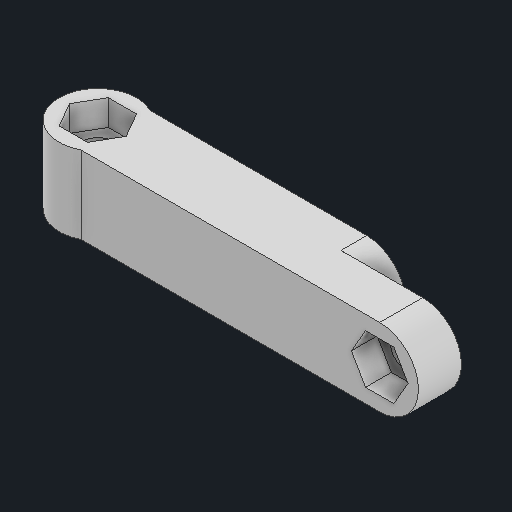
# Autodesk Inventor part: L1
Saved by Autodesk Inventor 2023.4 (Build 274418000, 418)
## iProperties
Created: 2024-10-16
Part Number: L1
Material: Ogólny
Document SubType Name: Modeling
Designer: kamil
Density: 1 g/cm^3
Appearance: Domyślna
Author: kamil
Autodesk Inventor part; units mm, degrees
ref_plane "YZ Plane" through (0, 0, 0) normal (1, 0, 0) x (0, 1, 0)
ref_plane "Płaszczyzna konstrukcyjna2" through (-16.0063, -4.5, 5) normal (0, 0, 1) x (1, 0, 0)
sketch "Szkic1" plane through (0, 0, 0) normal (0, 0, 1) x (1, 0, 0)
  circle A0 centre (-21, 0) radius 1.75 projected
  arc A1 (-11.0125, 4.5) -> (-15.9781, 0.0856) centre (-11.0125, -0.5) ccw projected
  line L0 (-21, 4.5) -> (-11.0125, 4.5) projected
  arc A2 (-21, 4.5) -> (-21, -4.5) centre (-21, 0) ccw projected
  line L1 (-11.0628, -4.5) -> (-21, -4.5) projected
  arc A3 (-15.9446, -0.5811) -> (-11.0628, -4.5) centre (-11.0628, 0.5) ccw projected
  line L2 (-21, 0) -> (-57.75, 0)
  line L3 (-21, 0) -> (-57.75, 0) construction
  line L4 (-21, -4.5) -> (-57.75, -4.5)
  line L5 (-57.75, 4.5) -> (-21, 4.5)
  arc A4 (-21, -4.5) -> (-21, 4.5) centre (-21, 0) ccw
  arc A5 (-57.75, 4.5) -> (-57.75, -4.5) centre (-57.75, 0) ccw
  line L6 (-57.75, 4.5) -> (-57.75, -4.5)
  arc A6 (-15.9781, 0.0856) -> (-15.9446, -0.5811) centre (-13.9919, -0.1486) ccw projected
  point P0 (0, 0)
  point P1 (-39.375, 0)
  dimension "d0" = 36.75
  constraints: 12 end point, 4 point on circle, 4 tangent, 2 centre point, 2 parallel, 1 collinear, 1 midpoint, 1 vertical
  measures "d0" distance of L2.start L2.end
extrude "Wyciągnięcie proste1" add sketch "Szkic1" along normal up to surface (5 mm away) contours A2 A4 | A2 L4 L6 L2 | L2 L6 L5 A2
sketch "Szkic2" plane through (0, 0, 0) normal (0, 0, -1) x (-1, 0, 0)
  line L0 (21, 4.5) -> (57.75, 4.5) projected
  arc A0 (21, 4.5) -> (21, -4.5) centre (21, 0) ccw projected
  line L1 (57.75, -4.5) -> (21, -4.5) projected
  line L2 (57.75, 4.5) -> (57.75, -4.5) projected
  circle A1 centre (21, 0) radius 1.75 projected
  arc A2 (21, -4.5) -> (21, 4.5) centre (21, 0) ccw projected
  circle A3 centre (21, 0) radius 5
  point P0 (0, 0)
  point P1 (23.1794, 4.5)
  point P2 (23.1794, -4.5)
  dimension "d3" = 10
  constraints: 1 centre point, 1 coincident
  measures "d3" diameter of A3
ref_plane "Płaszczyzna konstrukcyjna1" through (-25.5, -4.5, -3) normal (0, 0, -1) x (0, 1, 0)
extrude "Wyciągnięcie proste2" add sketch "Szkic2" along normal up to surface (3 mm away) contours L0 L2 L1 A3
fillet "Zaokrąglenie1" radius 4.5 2 edges at (-23.1794, -4.5, -1.5) (-23.1794, 4.5, -1.5)
sketch "Szkic4" plane through (-57.75, 4.5, 5) normal (0, 1, 0) x (1, 0, 0)
  line L0 (0, 8) -> (0, 0) projected
  circle A0 centre (0, 4) radius 1.75
  circle A1 centre (0, 4) radius 4
  point P0 (57.75, 5)
  point P1 (0, 2.25)
  point P2 (0, 5.75)
  dimension "d15" = 3.5
  constraints: 1 centre point, 1 coincident, 1 midpoint, 3 other
  measures "d15" diameter of A0
extrude "Wyciągnięcie proste6" add sketch "Szkic4" against normal up to surface (9 mm away) contours L0 A0 A1 picked at (-0.4587, 0.8057)
extrude "Wyciągnięcie proste7" cut sketch "Szkic4" against normal through all contours A0 L0 picked at (0.2531, 4.5256)
sketch "Szkic5" plane through (-30.5, 0, -3) normal (0, 0, -1) x (-1, 0, 0)
  arc A0 (0, 4.5) -> (0, -4.5) centre (0, 0) ccw projected
  line L0 (27.25, -4.5) -> (0, -4.5) projected
  line L1 (27.25, 4.5) -> (27.25, -4.5) projected
  line L2 (0, 4.5) -> (27.25, 4.5) projected
  line L3 (29, -4.5) -> (29, 4.5) projected
  line L4 (25.5, -4.5) -> (25.5, 4.5) projected
  line L5 (23.5, -4.5) -> (23.5, 4.5)
  arc A1 (0, 2.5) -> (0, -2.5) centre (0, 0) ccw
  line L6 (0, 2.5) -> (25.25, 2.5)
  line L7 (25.25, 2.5) -> (25.25, -2.5)
  line L8 (25.25, -2.5) -> (0, -2.5)
  point P0 (-30.5, 0)
  point P1 (23.5, -2.5)
  point P2 (23.5, 2.5)
  dimension "d20" = 2
  dimension "d21" = 2
  constraints: 8 end point, 2 point on circle, 1 centre point, 1 parallel, 3 other
  measures "d20" distance between parallel lines of L4 L5
  measures "d21" distance between parallel lines of L0 L8
extrude "Wyciągnięcie proste8" cut sketch "Szkic5" against normal up to surface (3 mm away) contours L5 L8 A1 L6
fillet "Zaokrąglenie2" radius 2 2 edges at (-54, 2.5, -1.5) (-54, -2.5, -1.5)
sketch "Szkic6" plane through (-21, 0, 5) normal (0, 0, 1) x (1, 0, 0)
  circle A0 centre (0, 0) radius 1.75 projected
  circle A1 centre (0, 0) radius 2.85
  line L0 (1.6454, 2.85) -> (3.2909, 0)
  line L1 (3.2909, 0) -> (1.6454, -2.85)
  line L2 (1.6454, -2.85) -> (-1.6454, -2.85)
  line L3 (-1.6454, -2.85) -> (-3.2909, 0)
  line L4 (-3.2909, 0) -> (-1.6454, 2.85)
  line L5 (-1.6454, 2.85) -> (1.6454, 2.85)
  point P0 (21, 0)
  point P1 (0, 2.85)
  dimension "d25" = 5.7
  constraints: 12 end point, 2 coincident, 1 midpoint, 1 vertical alignment, 15 other
extrude "Wyciągnięcie proste9" cut sketch "Szkic6" against normal blind 3 contours A0 | A1 | A1 L0 L1 | A1 L5 L0 | L1 L2 A1 | A1 L4 L5 | L2 L3 A1 | A1 L3 L4
sketch "Szkic7" plane through (-21, 4.5, 5) normal (0, 1, 0) x (1, 0, 0)
  circle A0 centre (-36.75, 4) radius 1.75 projected
  circle A1 centre (-36.75, 4) radius 2.85
  circle A2 centre (-36.75, 4) radius 1.75 projected
  line L0 (-35.1046, 6.85) -> (-33.4591, 4)
  line L1 (-33.4591, 4) -> (-35.1046, 1.15)
  line L2 (-35.1046, 1.15) -> (-38.3954, 1.15)
  line L3 (-38.3954, 1.15) -> (-40.0409, 4)
  line L4 (-40.0409, 4) -> (-38.3954, 6.85)
  line L5 (-38.3954, 6.85) -> (-35.1046, 6.85)
  point P0 (21, 5)
  point P1 (-36.75, 6.85)
  dimension "d28" = 5.7
  constraints: 12 end point, 2 coincident, 1 midpoint, 1 vertical alignment, 15 other
extrude "Wyciągnięcie proste10" cut sketch "Szkic7" against normal blind 3 contours A0 | A1 | A1 L0 L1 | A1 L5 L0 | L1 L2 A1 | A1 L4 L5 | L2 L3 A1 | A1 L3 L4
sketch "Szkic8" plane through (-21, -4.5, 0) normal (0, -1, 0) x (1, 0, 0)
  circle A0 centre (-36.75, 1) radius 1.75 projected
  circle A1 centre (-36.75, 1) radius 4.5
  arc A2 (-36.75, 5) -> (-36.75, -3) centre (-36.75, 1) ccw projected
  circle A3 centre (-36.75, 1) radius 1.75 projected
  arc A4 (-36.75, 5) -> (-36.75, -3) centre (-36.75, 1) ccw projected
  line L0 (-36.75, -3) -> (-9.5, -3) projected
  line L1 (-9.5, 0) -> (-9.5, -3) projected
  line L2 (-9.5, 0) -> (0, 0) projected
  line L3 (0, 0) -> (0, 5) projected
  line L4 (0, 5) -> (-36.75, 5) projected
  point P0 (21, 0)
  point P1 (-34.6884, 5)
  point P2 (-34.6884, -3)
  dimension "d31" = 9
  constraints: 1 centre point, 1 coincident
  measures "d31" diameter of A1
extrude "Wyciągnięcie proste11" add sketch "Szkic8" against normal up to surface (9 mm away) contours L4 A2 L0 A1 picked at (-35.7134, 5.1254)
